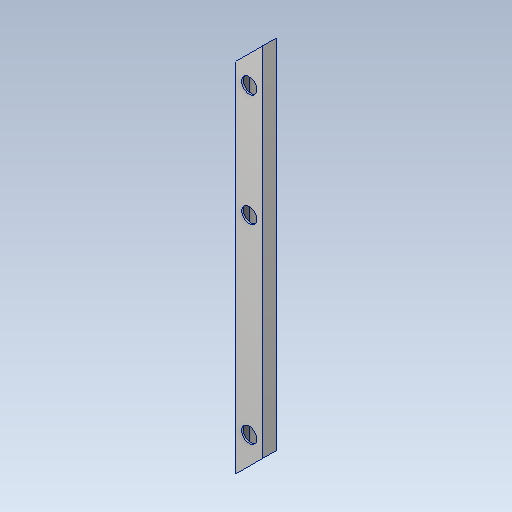
# Autodesk Inventor part: AngleBrace.ver2-1111-2020
Saved by Autodesk Inventor 2021 (Build 250183000, 183)
## iProperties
Created: 2020-01-19
Part Number: AngleBrace.ver2-1111-2020
Material: Aluminum 6061
Document SubType Name: Modeling
Designer: JMHal
Density: 2.7 g/cm^3
Appearance: Aluminum - Flat
Author: JMHal
Autodesk Inventor part; units mm, degrees
ref_plane "YZ Plane" through (0, 0, 0) normal (1, 0, 0) x (0, 1, 0)
ref_plane "XZ Plane" through (0, 0, 0) normal (0, 1, 0) x (-1, 0, 0)
ref_plane "XY Plane" through (0, 0, 0) normal (0, 0, 1) x (1, 0, 0)
sketch "Sketch1" plane through (0, 0, 0) normal (0, 1, 0) x (-1, 0, 0)
  line L0 (0, 0) -> (50.8, 0)
  line L1 (50.8, 0) -> (50.8, -25.4)
  line L2 (50.8, -25.4) -> (0, -25.4)
  line L3 (0, -25.4) -> (0, 0)
  line L4 (47.625, -22.225) -> (47.625, -3.175)
  line L5 (47.625, -3.175) -> (3.175, -3.175)
  line L6 (3.175, -3.175) -> (3.175, -22.225)
  line L7 (3.175, -22.225) -> (47.625, -22.225)
  dimension "d0" = 50.8
  dimension "d1" = 25.4
  dimension "d2" = 3.175
  constraints: 16 end point, 4 parallel, 2 perpendicular, 1 horizontal, 3 other
  measures "d0" distance of L1.end L2.end
  measures "d1" distance of L0.end L1.end
  measures "d2" distance between parallel lines of L1 L4
extrude "Extrusion1" add sketch "Sketch1" along normal blind 886.206
sketch "Sketch2" plane through (-50.8, 0, 0) normal (0, 0, 1) x (1, 0, 0)
  line L0 (50.8, 0) -> (0, 0) projected
  line L1 (50.8, 0) -> (50.8, 886.206) projected
  line L2 (0, 886.206) -> (50.8, 886.206) projected
  line L3 (0, 0) -> (0, 886.206) projected
  line L4 (0, 0) -> (50.8, 0) projected
  line L5 (50.8, 0) -> (0, 56.4191)
  line L6 (0, 56.4191) -> (50.8, 56.4191)
  line L7 (50.8, 56.4191) -> (50.8, 0)
  line L8 (50.8, 0) -> (0, 0)
  line L9 (0, 0) -> (0, 56.4191)
  line L10 (0, 56.4191) -> (50.8, 0)
  line L11 (0, 56.4191) -> (21.859, 0)
  line L12 (47.625, 0) -> (3.175, 0) projected
  dimension "d5" = 48
  constraints: 14 end point, 2 parallel, 2 point on line, 1 horizontal, 1 perpendicular
  measures "d5" angle of L5 L0
extrude "Extrusion2" cut sketch "Sketch2" against normal blind 914.4 contours L0 L11 L5 | L11 L0 L3
sketch "Sketch3" plane through (-50.8, 886.206, 0) normal (0, 0, 1) x (1, 0, 0)
  line L0 (0, -829.7869) -> (50.8, -886.206) projected
  line L1 (50.8, -886.206) -> (50.8, 0) projected
  line L2 (0, 0) -> (50.8, 0) projected
  line L3 (0, -829.7869) -> (0, 0) projected
  line L4 (0, -829.7869) -> (50.8, -886.206) projected
  line L5 (0, -829.7869) -> (50.8, -778.9869)
  line L6 (50.8, -886.206) -> (50.8, 0) projected
  line L7 (0, -829.7869) -> (0, 0) projected
  line L8 (50.8, -886.206) -> (0, -886.206)
  line L9 (0, -886.206) -> (0, -923.3654)
  line L10 (0, -923.3654) -> (50.8, -923.3654)
  line L11 (50.8, -923.3654) -> (50.8, -886.206)
  dimension "d8" = 93
  constraints: 10 end point, 4 point on line, 2 parallel, 1 horizontal, 1 perpendicular
  measures "d8" angle of L0 L5
extrude "Extrusion3" cut sketch "Sketch3" against normal blind 25.4 contours L5 L1 L0
sketch "Sketch4" plane through (-50.8, 886.206, 0) normal (0, 0, 1) x (1, 0, 0)
  line L0 (0, -829.7869) -> (50.8, -778.9869) projected
  line L1 (50.8, -778.9869) -> (50.8, 0) projected
  line L2 (0, 0) -> (50.8, 0) projected
  line L3 (0, -829.7869) -> (0, 0) projected
  line L4 (0, 0) -> (50.8, 0) projected
  line L5 (0, 0) -> (50.8, 0)
  line L6 (50.8, 0) -> (50.8, -221.7928)
  line L7 (50.8, -221.7928) -> (0, -221.7928)
  line L8 (0, -221.7928) -> (0, 0)
  line L9 (0, -829.7869) -> (0, 0) projected
  line L10 (0, 0) -> (50.8, -50.8)
  line L11 (50.8, 0) -> (0, 0)
  line L12 (0, 0) -> (0, -56.4191)
  line L13 (0, -56.4191) -> (50.8, -56.4191)
  line L14 (50.8, -56.4191) -> (50.8, 0)
  point P0 (50.8, -886.206)
  dimension "d11" = 221.7928
  dimension "d12" = 45
  dimension "d13" = 56.4191
  constraints: 18 end point, 4 parallel, 3 point on line, 2 horizontal, 2 perpendicular
  measures "d11" distance between parallel lines of L7 L2
  measures "d12" angle of L2 L10
  measures "d13" distance between parallel lines of L13 L2
extrude "Extrusion4" cut sketch "Sketch4" against normal blind 25.4 contours L2 L1 L10
sketch "Sketch8" plane through (-50.8, 56.4191, 0) normal (0, 0, 1) x (1, 0, 0)
  line L0 (50.8, 778.9869) -> (0, 829.7869) projected
  line L1 (0, 0) -> (0, 829.7869) projected
  line L2 (0, 0) -> (50.8, 50.8) projected
  line L3 (50.8, 50.8) -> (50.8, 778.9869) projected
  line L4 (0, 797.6016) -> (50.8, 746.8016)
  point P0 (50.8, -56.4191)
  dimension "d24" = 22.7584
  constraints: 2 end point, 2 point on line
  measures "d24" distance between parallel lines of L0 L4
extrude "Extrusion8" cut sketch "Sketch8" against normal blind 25.4 contours L3 L4 L1 L0
sketch "Sketch9" plane through (-50.8, 56.4191, 0) normal (0, 0, 1) x (1, 0, 0)
  line L0 (50.8, 746.8016) -> (0, 797.6016) projected
  line L1 (0, 0) -> (0, 797.6016) projected
  line L2 (0, 0) -> (50.8, 50.8) projected
  line L3 (50.8, 50.8) -> (50.8, 746.8016) projected
  line L4 (0, 0) -> (0, 797.6016) projected
  line L5 (0, 58.228) -> (50.8, 109.028)
  line L6 (50.8, 50.8) -> (50.8, 746.8016) projected
  line L7 (0, 0) -> (50.8, 50.8) projected
  point P0 (50.8, -56.4191)
  dimension "d27" = 41.1734
  constraints: 2 end point, 2 point on line, 1 parallel
  measures "d27" distance between parallel lines of L5 L2
extrude "Extrusion9" cut sketch "Sketch9" against normal blind 25.4 contours L3 L2 L1 L5
sketch "Sketch10" plane through (-50.8, 114.6471, 0) normal (0, 0, 1) x (1, 0, 0)
  line L0 (0, 0) -> (50.8, 50.8) projected
  line L1 (50.8, 50.8) -> (50.8, 688.5737) projected
  line L2 (50.8, 688.5737) -> (0, 739.3737) projected
  line L3 (0, 0) -> (0, 739.3737) projected
  point P0 (50.8, -114.6471)
  point P1 (25.4, 76.2)
hole "Hole1" at (-25.4, 190.8471, 0) direction (0, 0, -1) diameter 28.575 end through all
sketch "Sketch11" plane through (-50.8, 114.6471, 0) normal (0, 0, 1) x (1, 0, 0)
  circle A0 centre (25.4, 76.2) radius 14.2875 projected
  line L0 (0, 0) -> (50.8, 50.8) projected
  line L1 (50.8, 50.8) -> (50.8, 688.5737) projected
  line L2 (50.8, 688.5737) -> (0, 739.3737) projected
  line L3 (0, 0) -> (0, 739.3737) projected
  point P0 (50.8, -114.6471)
  point P1 (25.4, 431.8)
  dimension "d37" = 355.6
  measures "d37" distance of A0.centre point (25.4, 431.8)
hole "Hole2" at (-25.4, 546.4471, 0) direction (0, 0, -1) diameter 28.575 end through all
sketch "Sketch12" plane through (-50.8, 114.6471, 0) normal (0, 0, 1) x (1, 0, 0)
  circle A0 centre (25.4, 431.8) radius 14.2875 projected
  circle A1 centre (25.4, 76.2) radius 14.2875 projected
  line L0 (50.8, 50.8) -> (0, 0) projected
  line L1 (0, 0) -> (0, 739.3737) projected
  line L2 (0, 739.3737) -> (50.8, 688.5737) projected
  line L3 (50.8, 50.8) -> (50.8, 688.5737) projected
  line L4 (50.8, 50.8) -> (50.8, 688.5737) projected
  line L5 (50.8, 688.5737) -> (29.7688, 688.5737)
  line L6 (29.7688, 688.5737) -> (29.7688, 709.6049)
  line L7 (29.7688, 709.6049) -> (50.8, 709.6049)
  line L8 (50.8, 709.6049) -> (50.8, 688.5737)
  line L9 (50.8, 709.6049) -> (0, 658.8049)
  line L10 (0, 0) -> (0, 739.3737) projected
  line L11 (0, 658.8049) -> (50.8, 658.8049)
  line L12 (50.8, 658.8049) -> (50.8, 739.3737)
  line L13 (50.8, 739.3737) -> (0, 739.3737)
  line L14 (0, 739.3737) -> (0, 658.8049)
  line L15 (0, 739.3737) -> (50.8, 688.5737)
  line L16 (50.8, 709.6049) -> (29.7688, 688.5737)
  line L17 (50.8, 688.5737) -> (50.8, 709.6049)
  line L18 (29.7688, 688.5737) -> (50.8, 688.5737)
  point P0 (50.8, -114.6471)
  dimension "d45" = 21.0312
  dimension "d46" = 21.0312
  dimension "d47" = 50.8
  dimension "d48" = 80.5688
  dimension "d49" = 50.8
  constraints: 26 end point, 5 point on line, 4 parallel, 2 horizontal, 2 perpendicular
  measures "d45" distance of L6.end L7.end
  measures "d46" distance of L7.end L2.end
  measures "d47" horizontal distance of L7.end L9.end
  measures "d48" distance of L11.end L12.end
  measures "d49" distance of L12.end L13.end
extrude "Extrusion10" add sketch "Sketch12" against normal blind 25.4 contours L5 L9 L2 | L2 L9 L8
extrude "Extrusion11" cut sketch "Sketch12" against normal blind 25.4 contours L1 L2 L6 L9 | L13 L12 L7 L2
sketch "Sketch14" plane through (0, 165.4471, -25.4) normal (0, 0, -1) x (-1, 0, 0)
  circle A0 centre (25.4, 381) radius 14.2875 projected
  circle A1 centre (25.4, 25.4) radius 14.2875 projected
  line L0 (50.8, 608.0049) -> (21.0312, 637.7737) projected
  line L1 (21.0312, 637.7737) -> (21.0312, 658.8049) projected
  line L2 (21.0312, 658.8049) -> (10.5156, 648.2893) projected
  line L3 (10.5156, 648.2893) -> (0, 658.8049) projected
  line L4 (0, 0) -> (0, 658.8049) projected
  line L5 (0, 0) -> (50.8, -50.8) projected
  line L6 (50.8, -50.8) -> (50.8, 608.0049) projected
  line L7 (10.5156, 648.2893) -> (21.0312, 637.7737)
  line L8 (21.0312, 637.7737) -> (47.625, 611.1799) projected
  line L9 (21.0312, 637.7737) -> (21.0312, 658.8049) projected
  line L10 (21.0312, 658.8049) -> (21.0312, 637.7737)
  line L11 (10.5156, 648.2893) -> (21.0312, 658.8049)
  point P0 (0, -165.4471)
  constraints: 6 end point, 2 point on line
extrude "Extrusion12" cut sketch "Sketch14" against normal through all contours L7 L2 L1
sketch "Sketch15" plane through (0, 0, 0) normal (0, 1, 0) x (-1, 0, 0)
  line L0 (47.625, -22.225) -> (3.175, -22.225) projected
  line L1 (3.175, -3.175) -> (47.625, -3.175) projected
  line L2 (47.625, -3.175) -> (47.625, -22.225) projected
  line L3 (3.175, -22.225) -> (3.175, -3.175) projected
  point P0 (0, 0)
extrude "Extrusion13" cut sketch "Sketch15" along normal blind 2540
sketch "Sketch16" plane through (0, 165.4471, -25.4) normal (0, 0, -1) x (-1, 0, 0)
  line L0 (50.8, 608.0049) -> (0, 658.8049) projected
  line L1 (0, 0) -> (0, 658.8049) projected
  line L2 (0, 0) -> (50.8, -50.8) projected
  line L3 (50.8, -50.8) -> (50.8, 608.0049) projected
  circle A0 centre (25.4, 25.4) radius 14.2875 projected
  circle A1 centre (25.4, 381) radius 14.2875 projected
  line L4 (50.8, 608.0049) -> (-0.2406, 608.0049)
  line L5 (11.1125, 647.6924) -> (15.4769, 652.0568)
  line L6 (50.8, 616.7337) -> (-0.2406, 667.7743)
  line L7 (47.625, 611.1799) -> (3.175, 655.6299) projected
  line L8 (0, 658.8049) -> (0, 667.5337)
  line L9 (0, 658.8049) -> (50.8, 608.0049) projected
  line L10 (50.8, 608.0049) -> (50.8, 616.7337)
  line L11 (0, 658.8049) -> (50.8, 608.0049)
  point P0 (0, -165.4471)
  dimension "d58" = 6.1722
  dimension "d59" = 90
  dimension "d60" = 8.7288
  constraints: 12 end point, 4 point on line, 1 collinear, 1 horizontal, 1 parallel
  measures "d58" distance of L5.start L5.end
  measures "d59" angle of L0 L5
  measures "d60" distance of L0.start L6.start
extrude "Extrusion14" add sketch "Sketch16" against normal blind 25.4 contours L0 L5 L6 L10 | L0 L8 L6 L5
sketch "Sketch17" plane through (0, 0, 0) normal (0, 1, 0) x (-1, 0, 0)
  line L0 (47.625, -3.175) -> (3.175, -3.175) projected
  line L1 (47.625, -22.225) -> (47.625, -3.175) projected
  line L2 (47.625, -22.225) -> (3.175, -22.225) projected
  line L3 (3.175, -22.225) -> (3.175, -3.175) projected
  point P0 (0, 0)
extrude "Extrusion15" cut sketch "Sketch17" along normal blind 2540
sketch "Sketch18" plane through (-50.8, 114.6471, 0) normal (0, 0, 1) x (1, 0, 0)
  circle A0 centre (25.4, 431.8) radius 14.2875 projected
  circle A1 centre (25.4, 431.8) radius 14.2875
  circle A2 centre (25.4, 641.35) radius 14.2875
  point P0 (50.8, -114.6471)
  dimension "d65" = 28.575
  dimension "d66" = 209.55
  constraints: 2 centre point, 1 coincident
  measures "d65" diameter of A2
  measures "d66" distance of A0.centre A2.centre
extrude "Extrusion16" cut sketch "Sketch18" against normal blind 25.4 contours A2
body "Solid1"
